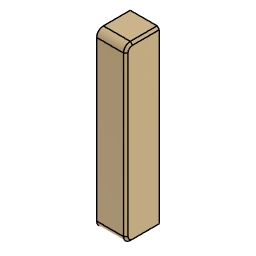
Tampa janela Emoções v2 (Autodesk Fusion 360 design; units mm, degrees)
Autodesk Fusion 360 part; units mm, degrees
sketch "Sketch1" plane through (0, 0, 0) normal (1, 0, 0) x (0, 1, 0)
  line L0 (0, 0) -> (-12, 0)
  arc A0 (-15, 3) -> (-12, 0) centre (-12, 3) ccw
  line L1 (-15, 3) -> (-15, 74)
  arc A1 (-12, 77) -> (-15, 74) centre (-12, 74) ccw
  line L2 (-12, 77) -> (0, 77)
  line L3 (0, 77) -> (0, 0)
  line L4 (0, 68.5) -> (-11, 68.5)
  line L5 (-11, 68.5) -> (-11, 8.5)
  line L6 (-11, 8.5) -> (0, 8.5)
  line L7 (-11, 38.5) -> (-15, 38.5) construction
  dimension "d1" = 60
  dimension "d2" = 77
  dimension "d3" = 3
  dimension "d4" = 15
  dimension "d5" = 11
  constraint coincident L0.start L3.end
  constraint horizontal L0
  constraint tangent L0 A0
  constraint perpendicular L0 L1
  constraint tangent L1 A1
  constraint perpendicular L1 L2
  constraint perpendicular L0 L3
  constraint tangent A1 L2
  constraint tangent A0 L1
  constraint coincident L3 L4.start
  constraint perpendicular L3 L4
  constraint perpendicular L4 L5
  constraint perpendicular L3 L6
  constraint midpoint L5 L7.start
  constraint midpoint L1 L7.end
  constraint horizontal L7
  constraint coincident L3 L6.end
  constraint equal A0 A1
  measures "d1" distance of L4.end L5.end
  measures "d2" distance of L2.end L0.start
  measures "d3" radius of A1
  measures "d4" distance of L1 L3
  measures "d5" distance of L4.start L4.end
extrude "Extrude1" add sketch "Sketch1" against normal blind 10 contours L0 A0 L1 A1 L2 L3 L4 L5 L6
extrude "Extrude2" add sketch "Sketch1" along normal blind 3
fillet "Fillet1" radius 1 2 edges at (-5, -11, 68.5) (-5, -11, 8.5)
chamfer "Chamfer1" distance 1 angle 45 10 edges at (3, -6, 77) (3, -14.1213, 76.1213) (3, -15, 38.5) (3, -14.1213, 0.8787) (3, -6, 0) (0, -5, 68.5) (0, -10.7071, 68.2071) (0, -11, 38.5) (0, -10.7071, 8.7929) (0, -5, 8.5)
